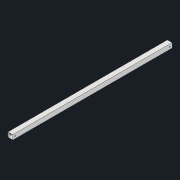
# Autodesk Inventor part: Side Bar
Saved by Autodesk Inventor 2022 (Build 260153000, 153)
## iProperties
Created: 2022-09-10
Part Number: Side Bar
Material: Generic
Document SubType Name: Modeling
Designer: robpl
Density: 1 g/cm^3
Appearance: Default
Author: robpl
Autodesk Inventor part; units mm, degrees
ref_plane "YZ Plane" through (0, 0, 0) normal (1, 0, 0) x (0, 1, 0)
ref_plane "XZ Plane" through (0, 0, 0) normal (0, 1, 0) x (-1, 0, 0)
ref_plane "XY Plane" through (0, 0, 0) normal (0, 0, 1) x (1, 0, 0)
sketch "Sketch1" plane through (0, 0, 0) normal (0, 0, 1) x (1, 0, 0)
  line L0 (0, 0) -> (25, 0)
  line L1 (25, 0) -> (25, 25)
  line L2 (25, 25) -> (0, 25)
  line L3 (0, 25) -> (0, 0)
  line L4 (23.5, 23.5) -> (23.5, 1.5)
  line L5 (23.5, 1.5) -> (1.5, 1.5)
  line L6 (1.5, 1.5) -> (1.5, 23.5)
  line L7 (1.5, 23.5) -> (23.5, 23.5)
  dimension "d0" = 25
  dimension "d1" = 25
  dimension "d2" = 1.5
  constraints: 16 end point, 4 parallel, 2 perpendicular, 1 horizontal, 3 other
  measures "d0" distance of L2.end L1.end
  measures "d1" distance of L1.end L0.end
  measures "d2" distance between parallel lines of L1 L4
extrude "Extrusion1" add sketch "Sketch1" along normal blind 850
sketch "Sketch2" plane through (0, 0, 0) normal (1, 0, 0) x (0, 0, -1)
  line L0 (0, 0) -> (0, 25) projected
  line L1 (-850, 0) -> (-850, 25) projected
  point P0 (-837.5, 12.5)
  point P1 (-12.5, 12.5)
  dimension "d5" = 12.5
  dimension "d6" = 12.5
  dimension "d7" = 12.5
  constraints: 1 horizontal alignment
  measures "d5" distance from line of L0 point (-12.5, 12.5)
  measures "d6" horizontal distance of point (-12.5, 12.5) L0.start
  measures "d7" distance from line of L1 point (-837.5, 12.5)
hole "Hole1" at (0, 12.5, 837.5) at (0, 12.5, 12.5) direction (1, 0, 0) diameter 6 end through all counterbore diameter 11 counterbore depth 5
equation "\"d6\" = d5"
body "Solid1"
